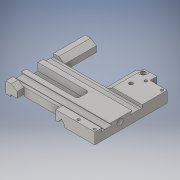
# Autodesk Inventor part: saddle
Saved by Autodesk Inventor 2016 (Build 200138000, 138)
## iProperties
Created: 2017-02-14
Part Number: saddle
Material: Generic
Document SubType Name: Modeling
Designer: M228544
Density: 1 g/cm^3
Appearance: Default
Author: M228544
Autodesk Inventor part; units mm, degrees
ref_plane "YZ Plane" through (0, 0, 0) normal (1, 0, 0) x (0, 1, 0)
ref_plane "XZ Plane" through (0, 0, 0) normal (0, 1, 0) x (-1, 0, 0)
ref_plane "XY Plane" through (0, 0, 0) normal (0, 0, 1) x (1, 0, 0)
sketch "Sketch1" plane through (0, 0, 0) normal (0, 1, 0) x (-1, 0, 0)
  line L0 (0, 0) -> (-384, 0)
  line L1 (-384, 0) -> (-384, -343)
  line L2 (-384, -343) -> (0, -343)
  line L3 (0, -343) -> (0, 0)
  dimension "d0" = 384
  dimension "d1" = 343
  constraints: 8 end point, 2 parallel, 1 horizontal, 1 perpendicular
  measures "d0" distance of L2.end L1.end
  measures "d1" distance of L1.end L0.end
extrude "Extrusion1" add sketch "Sketch1" along normal blind 48.5
sketch "Sketch3" plane through (384, 0, 0) normal (1, 0, 0) x (0, 0, -1)
  line L0 (0, 0) -> (343, 0) projected
  line L1 (0, 0) -> (0, 48.5) projected
  line L2 (343, 0) -> (343, 48.5) projected
  line L3 (30, 48.5) -> (65, 48.5)
  line L4 (30, 48.5) -> (30, 37)
  line L5 (65, 48.5) -> (74.6496, 37)
  line L6 (43, 37) -> (74.6496, 37)
  line L7 (30, 37) -> (30, 35)
  line L8 (30, 35) -> (43, 35)
  line L9 (43, 35) -> (43, 37)
  dimension "d23" = 35
  dimension "d37" = 2
  dimension "d38" = 13
  constraints: 14 end point, 2 perpendicular, 1 horizontal, 1 vertical
  measures "d23" distance of L3.start L3.end
  measures "d37" distance of L4.end L7.end
  measures "d38" distance of L7.end L8.end
extrude "Extrusion2" cut sketch "Sketch3" against normal through all
sketch "Sketch7" plane through (384, 0, 0) normal (1, 0, 0) x (0, 0, -1)
  line L0 (65, 48.5) -> (343, 48.5) projected
  line L1 (65, 48.5) -> (161, 48.5)
  line L2 (161, 48.5) -> (174.2196, 48.5) construction
  line L3 (161, 48.5) -> (205, 48.5)
  line L4 (0, 0) -> (343, 0) projected
  line L5 (151.3504, 37) -> (192, 37)
  line L6 (205, 37) -> (205, 48.5)
  line L7 (161, 48.5) -> (151.3504, 37)
  line L8 (161, 48.5) -> (183.0653, 48.5) construction
  line L9 (205, 37) -> (205, 35)
  line L10 (205, 35) -> (192, 35)
  line L11 (192, 35) -> (192, 37)
  dimension "d27" = 96
  dimension "d29" = 44
  dimension "d32" = 130
  constraints: 20 end point, 3 horizontal, 3 perpendicular, 2 point on line, 1 vertical
  measures "d27" distance of L0.start L1.end
  measures "d29" distance of L1.end L3.end
  measures "d32" angle of L7 L8
extrude "Extrusion3" cut sketch "Sketch7" against normal through all
sketch "Sketch8" plane through (0, 48.5, 0) normal (0, 1, 0) x (1, 0, 0)
  line L0 (310, 343) -> (310, 316)
  line L1 (313, 313) -> (384, 313)
  line L2 (384, 0) -> (384, 343) projected
  line L3 (384, 313) -> (384, 343)
  line L4 (384, 343) -> (310, 343)
  line L5 (384, 343) -> (0, 343) projected
  arc A0 (310, 316) -> (313, 313) centre (313, 316) ccw
  point P0 (0, 0)
  point P1 (310, 313)
  dimension "d43" = 30
  dimension "d46" = 3
  constraints: 8 end point, 2 collinear, 2 point on circle, 2 point on line, 2 tangent, 1 centre point
  measures "d43" distance of L0.start point (310, 313)
  measures "d46" radius of A0
extrude "Extrusion4" cut sketch "Sketch8" against normal through all
sketch "Sketch9" plane through (0, 0, -343) normal (0, 0, -1) x (-1, 0, 0)
  line L0 (-215, 7) -> (-225, 7)
  line L1 (-255, 7) -> (-255, 0)
  line L2 (-255, 7) -> (-240, 24.8763)
  line L3 (-225, 7) -> (-240, 24.8763)
  line L4 (-215, 7) -> (-215, 0)
  line L5 (-255, 0) -> (-215, 0)
  dimension "d50" = 10
  constraints: 12 end point
  measures "d50" distance of L0.start L0.end
extrude "Extrusion5" cut sketch "Sketch9" against normal through all
sketch "Sketch10" plane through (0, 48.5, 0) normal (0, 1, 0) x (1, 0, 0)
  line L0 (215, 343) -> (215, 0) projected
  line L1 (215, 343) -> (215, 0) projected
  line L2 (310, 343) -> (0, 343) projected
  line L3 (384, 151.3504) -> (0, 151.3504) projected
  line L4 (215, 343) -> (48, 343)
  line L5 (48, 343) -> (48, 204)
  line L6 (48, 204) -> (215, 204)
  line L7 (215, 204) -> (215, 343)
  point P0 (0, 0)
  dimension "d58" = 167
  dimension "d59" = 139
  constraints: 8 end point, 2 parallel, 1 horizontal, 1 perpendicular
  measures "d58" distance of L6.end L5.end
  measures "d59" distance of L5.end L4.end
extrude "Extrusion6" cut sketch "Sketch10" against normal through all
sketch "Sketch11" plane through (0, 0, -343) normal (0, 0, -1) x (-1, 0, 0)
  line L0 (-20, 0) -> (-20, 7)
  line L1 (-20, 7) -> (-48, 7)
  line L2 (-48, 0) -> (-48, 7)
  line L3 (-48, 0) -> (-20, 0)
  dimension "d65" = 7
  constraints: 8 end point, 1 horizontal
  measures "d65" distance of L0.start L0.end
extrude "Extrusion7" cut sketch "Sketch11" against normal through all
sketch "Sketch12" plane through (0, 48.5, 0) normal (0, 1, 0) x (1, 0, 0)
  line L0 (221, 113) -> (221, 128)
  line L1 (211, 88) -> (0, 88)
  line L2 (211, 138) -> (0, 138)
  arc A0 (211, 88) -> (221, 98) centre (211, 98) ccw
  arc A1 (221, 128) -> (211, 138) centre (211, 128) ccw
  line L3 (221, 98) -> (221, 113)
  line L4 (0, 88) -> (0, 138)
  point P0 (384, 161)
  point P1 (221, 88)
  dimension "d72" = 10
  constraints: 10 end point, 4 point on circle, 3 tangent, 2 centre point, 2 point on line, 1 equal radius, 1 horizontal, 1 parallel, 1 perpendicular, 1 vertical
  measures "d72" radius of A0
extrude "Extrusion8" cut sketch "Sketch12" against normal blind 33
sketch "Sketch14" plane through (384, 0, 0) normal (1, 0, 0) x (0, 0, -1)
  circle A0 centre (109.1034, 31.5) radius 13.5
  line L0 (65, 48.5) -> (161, 48.5) projected
  point P0 (0, 0)
  dimension "d92" = 27
  dimension "d97" = 17
  constraints: 1 centre point
  measures "d92" diameter of A0
  measures "d97" distance from line of A0.centre L0
extrude "Extrusion10" cut sketch "Sketch14" against normal through all
sketch "Sketch17" plane through (0, 0, -343) normal (0, 0, -1) x (-1, 0, 0)
  line L0 (-23, 48.5) -> (-48, 32.2648)
  line L1 (-211, 15.5) -> (0, 15.5) projected
  line L2 (-48, 35) -> (-48, 7) projected
  line L3 (-48, 32.2648) -> (-48, 48.5)
  line L4 (-23, 48.5) -> (-48, 48.5)
  point P0 (0, 0)
  point P1 (0, 48.5)
  dimension "d98" = 23
  constraints: 6 end point, 1 point on line
  measures "d98" distance of point (0, 48.5) L0.start
extrude "Extrusion11" cut sketch "Sketch17" against normal up to surface (138 mm away)
sketch "Sketch19" plane through (310, 0, -343) normal (0, 0, -1) x (-1, 0, 0)
  line L0 (0, 48.5) -> (0, 0) projected
  line L1 (55, 46.5) -> (74.3713, 46.5) construction
  line L2 (55, 46.5) -> (95, 21.5052)
  line L3 (55, 46.5) -> (104.9882, 46.5) construction
  line L4 (55, 46.5) -> (55, 48.5)
  line L5 (55, 48.5) -> (95, 48.5)
  line L6 (89, 48.5) -> (99, 48.5) projected
  line L7 (95, 48.5) -> (95, 21.5052)
  line L8 (95, 7) -> (95, 48.5) projected
  point P0 (310, 0)
  dimension "d109" = 32
  constraints: 12 end point, 2 horizontal, 1 collinear, 1 point on line
  measures "d109" angle of L2 L3
extrude "Extrusion12" cut sketch "Sketch19" against normal up to surface (138 mm away)
sketch "Sketch25" plane through (0, 48.5, 0) normal (0, 1, 0) x (1, 0, 0)
  arc A0 (310, 316) -> (313, 313) centre (313, 316) ccw projected
  line L0 (265.5, 314) -> (255, 314)
  line L1 (255, 343) -> (255, 0) projected
  line L2 (310, 343) -> (255, 343) projected
  line L3 (280, 328.5) -> (280, 343)
  arc A1 (265.5, 314) -> (280, 328.5) centre (265.5, 328.5) ccw
  line L4 (280, 343) -> (255, 343)
  line L5 (255, 314) -> (255, 343)
  point P0 (0, 0)
  constraints: 8 end point, 2 collinear, 2 point on circle, 2 point on line, 1 centre point, 1 horizontal, 1 perpendicular, 1 tangent
extrude "Extrusion16" cut sketch "Sketch25" against normal blind 2
sketch "Sketch26" plane through (0, 46.5, 0) normal (0, 1, 0) x (1, 0, 0)
  line L0 (280, 343) -> (280, 328.5) projected
  circle A0 centre (265.5, 328.5) radius 9.5
  point P0 (0, 0)
  dimension "d136" = 19
  constraints: 1 centre point
  measures "d136" diameter of A0
extrude "Extrusion17" cut sketch "Sketch26" against normal blind 2
sketch "Sketch27" plane through (265.5, 44.5, -328.5) normal (0, 1, 0) x (1, 0, 0)
  circle A0 centre (0, 0) radius 6
  point P0 (-265.5, -328.5)
  dimension "d139" = 12
  constraints: 1 centre point
  measures "d139" diameter of A0
extrude "Extrusion18" cut sketch "Sketch27" against normal through all
sketch "Sketch28" plane through (0, 48.5, 0) normal (0, 1, 0) x (1, 0, 0)
  circle A0 centre (373, 302) radius 5.8
  circle A1 centre (303.4, 302) radius 5.8
  circle A2 centre (373, 11) radius 5.8
  circle A3 centre (303.4, 11) radius 5.8
  point P0 (0, 0)
  point P1 (384, 313)
  point P2 (384, 0)
  dimension "d146" = 11.6
  dimension "d149" = 11.6
  dimension "d152" = 11.6
  dimension "d155" = 11.6
  constraints: 4 centre point
  measures "d146" diameter of A0
  measures "d149" diameter of A1
  measures "d152" diameter of A2
  measures "d155" diameter of A3
extrude "Extrusion19" cut sketch "Sketch28" against normal through all
sketch "Sketch29" plane through (0, 48.5, 0) normal (0, 0, 1) x (1, 0, 0)
  line L0 (0, -48.5) -> (0, 0) projected
  line L1 (0, 0) -> (384, 0) projected
  line L2 (23, 0) -> (48, -16.2352) projected
  line L3 (23, 0) -> (48, -16.2352)
  line L4 (48, -48.5) -> (215, -48.5) projected
  line L5 (23, 0) -> (48, 0)
  line L6 (48, -16.2352) -> (48, 0)
  line L7 (384, -13.5) -> (0, -13.5) projected
  constraints: 6 end point, 1 collinear, 1 perpendicular, 1 point on line
extrude "Extrusion20" cut sketch "Sketch29" against normal up to surface (30 mm away) contours L7 L6 L2 | L2 L1 L6 L7
sketch "Sketch30" plane through (0, 0, 0) normal (0, 0, 1) x (1, 0, 0)
  line L0 (48, 48.5) -> (215, 48.5)
  line L1 (215, 48.5) -> (215, 0)
  line L2 (215, 0) -> (48, 0)
  line L3 (48, 0) -> (48, 48.5)
  point P0 (0, 0)
  constraints: 8 end point, 2 parallel, 1 horizontal, 1 perpendicular
extrude "Extrusion21" cut sketch "Sketch30" against normal up to surface (30 mm away)
sketch "Sketch32" plane through (0, 48.5, 0) normal (0, 1, 0) x (1, 0, 0)
  line L0 (275, 266) -> (283, 266) construction
  circle A0 centre (280.6569, 260.3431) radius 8
  point P0 (0, 0)
  point P1 (255, 343)
  dimension "d168" = 16
  constraints: 2 end point, 1 centre point, 1 horizontal
  measures "d168" diameter of A0
extrude "Extrusion22" cut sketch "Sketch32" against normal blind 10
body "Solid1"
